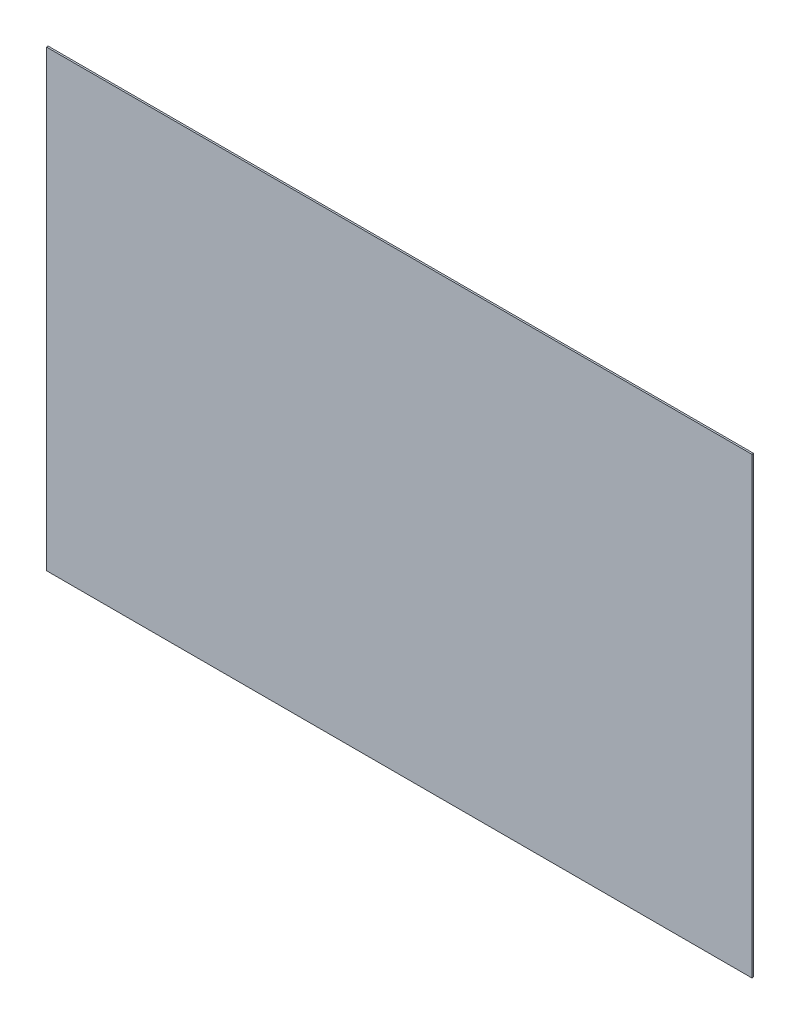
# Autodesk Inventor part: MATRYCA
Saved by Autodesk Inventor 2017 SP1 (Build 210196100, 196)
## iProperties
Created: 2021-03-14
Part Number: MATRYCA
Material: Poliwęglan dymiony
Document SubType Name: Modeling
Designer: Administrator
Density: 1.2 g/cm^3
Appearance: Poliwęglan - przydymiony
Author: Administrator
Autodesk Inventor part; units mm, degrees
ref_plane "YZ Plane" through (0, 0, 0) normal (1, 0, 0) x (0, 1, 0)
ref_plane "XZ Plane" through (0, 0, 0) normal (0, 1, 0) x (-1, 0, 0)
ref_plane "XY Plane" through (0, 0, 0) normal (0, 0, 1) x (1, 0, 0)
sketch "Szkic1" plane through (0, 0, 0) normal (0, 0, 1) x (1, 0, 0)
  line L0 (-210, 135) -> (210, 135)
  line L1 (210, 135) -> (210, -135)
  line L2 (210, -135) -> (-210, -135)
  line L3 (-210, -135) -> (-210, 135)
  dimension "d0" = 420
  dimension "d1" = 270
  constraints: 8 end point, 2 parallel, 1 horizontal, 1 perpendicular
  measures "d0" distance of L1.end L2.end
  measures "d1" distance of L0.end L1.end
extrude "Wyciągnięcie proste1" add sketch "Szkic1" along normal blind 1
